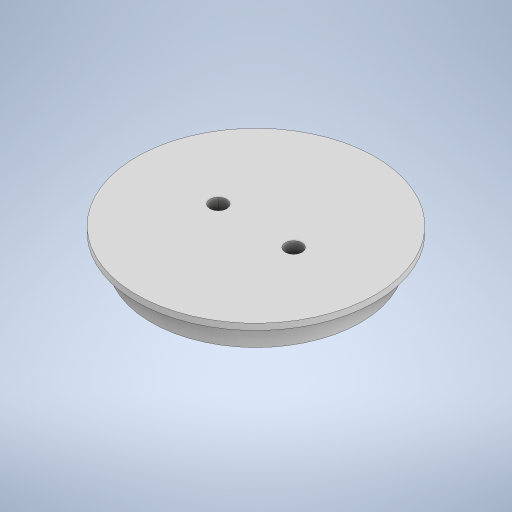
# Autodesk Inventor part: Wrist-Bearing Attachment
Saved by Autodesk Inventor 2023 (Build 270158000, 158)
## iProperties
Created: 2023-04-06
Part Number: Wrist-Bearing Attachment
Material: Generic
Document SubType Name: Modeling
Designer: adity
Density: 1 g/cm^3
Appearance: Default
Author: adity
Autodesk Inventor part; units mm, degrees
ref_plane "YZ Plane" through (0, 0, 0) normal (1, 0, 0) x (0, 1, 0)
ref_plane "XZ Plane" through (0, 0, 0) normal (0, 1, 0) x (-1, 0, 0)
sketch "Sketch1" plane through (0, 0, 0) normal (0, 1, 0) x (-1, 0, 0)
  circle A0 centre (0, 0) radius 13.5
  line L0 (0, 0) -> (9, 0)
  line L1 (0, 0) -> (-9, 0)
  circle A1 centre (-9, 0) radius 2
  circle A2 centre (9, 0) radius 2
  dimension "d0" = 27
  dimension "d1" = 9
  dimension "d2" = 9
  dimension "d3" = 4
  dimension "d4" = 4
  constraints: 4 end point, 3 centre point, 3 coincident, 2 horizontal
  measures "d0" diameter of A0
  measures "d1" distance of L0.start L0.end
  measures "d2" distance of L0.start L1.end
  measures "d3" diameter of A1
  measures "d4" diameter of A2
extrude "Extrusion1" add sketch "Sketch1" along normal blind 5
sketch "Sketch2" plane through (0, 5, 0) normal (0, 1, 0) x (1, 0, 0)
  circle A0 centre (0, 0) radius 25
  circle A1 centre (-9, 0) radius 2 projected
  circle A2 centre (9, 0) radius 2 projected
  circle A3 centre (-9, 0) radius 2 projected
  circle A4 centre (-9, 0) radius 2
  circle A5 centre (9, 0) radius 2 projected
  circle A6 centre (9, 0) radius 2
  dimension "d7" = 50
  constraints: 3 centre point, 3 coincident
  measures "d7" diameter of A0
extrude "Extrusion2" add sketch "Sketch2" along normal blind 6
sketch "Sketch3" plane through (0, 11, 0) normal (0, 1, 0) x (1, 0, 0)
  circle A0 centre (0, 0) radius 28.5
  circle A1 centre (-9, 0) radius 2 projected
  circle A2 centre (9, 0) radius 2 projected
  circle A3 centre (-9, 0) radius 2
  circle A4 centre (9, 0) radius 2 projected
  circle A5 centre (9, 0) radius 2
  dimension "d10" = 57
  constraints: 3 centre point, 3 coincident, 1 concentric
  measures "d10" diameter of A0
extrude "Extrusion4" add sketch "Sketch3" along normal blind 1.5
ref_plane "Work Plane1" through (-9, 0, 0) normal (0, 0, -1) x (0, 1, 0)
sketch "Sketch4" plane through (-9, 0, 0) normal (0, 0, -1) x (0, 1, 0)
  line L0 (0, 9) -> (5, 9)
  line L1 (5, -4.5) -> (5, 22.5) projected
  circle A0 centre (2.5, 9) radius 1.5
  dimension "d15" = 3
  constraints: 2 end point, 2 midpoint, 1 centre point
  measures "d15" diameter of A0
extrude "Extrusion5" cut sketch "Sketch4" against normal up to surface
body "Solid1"
